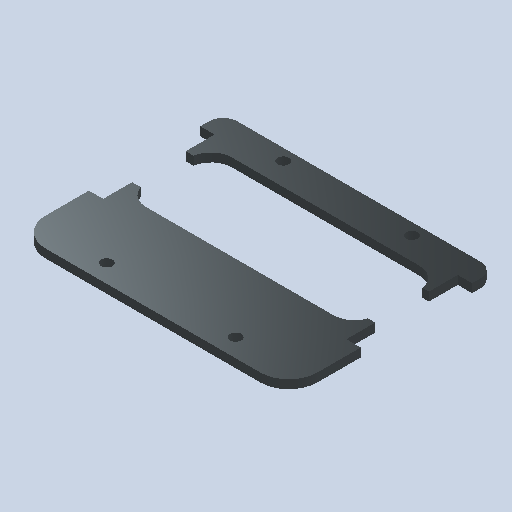
# Autodesk Inventor part: spacer
Saved by Autodesk Inventor 2022 (Build 260153000, 153)
## iProperties
Created: 2021-06-18
Part Number: spacer
Material: Iron, Gray
Document SubType Name: Modeling
Designer: benka
Density: 7.15 g/cm^3
Appearance: Iron Gray
Author: benka
Autodesk Inventor part; units mm, degrees
ref_plane "YZ Plane" through (0, 0, 0) normal (1, 0, 0) x (0, 1, 0)
ref_plane "XZ Plane" through (0, 0, 0) normal (0, 1, 0) x (-1, 0, 0)
ref_plane "XY Plane" through (0, 0, 0) normal (0, 0, 1) x (1, 0, 0)
sketch "Sketch1" plane through (0, 0, 0) normal (0, 1, 0) x (-1, 0, 0)
  arc A0 (-203.3189, -61.2561) -> (-210.2777, -66.3445) centre (-203.3189, -68.5586) ccw
  arc A1 (-130.8282, -66.3445) -> (-137.7869, -61.2561) centre (-137.7869, -68.5586) ccw
  arc A2 (-210.5383, -85.0627) -> (-203.3189, -91.2662) centre (-203.3189, -83.9637) ccw
  line L0 (-132.8206, -31.1315) -> (-207.8206, -31.1315)
  line L1 (-217.8206, -41.1315) -> (-217.8206, -56.2409)
  line L2 (-212.8206, -56.2409) -> (-217.8206, -56.2409) projected
  line L3 (-212.8206, -66.3445) -> (-212.8206, -56.2409) projected
  line L4 (-127.8206, -56.2409) -> (-127.8206, -66.3445) projected
  line L5 (-127.8206, -56.2409) -> (-122.8206, -56.2409) projected
  line L6 (-122.8206, -56.2409) -> (-122.8206, -41.1315)
  line L7 (-212.8206, -66.3445) -> (-210.2777, -66.3445)
  line L8 (-127.8206, -66.3445) -> (-130.8282, -66.3445)
  line L9 (-203.3189, -91.2662) -> (-137.7869, -91.2662)
  line L10 (-137.7869, -61.2561) -> (-203.3189, -61.2561) projected
  line L11 (-212.8208, -95.1662) -> (-212.8208, -85.0627) projected
  line L12 (-212.8208, -95.1662) -> (-217.8208, -95.1662) projected
  arc A3 (-217.8208, -98.1662) -> (-212.8208, -103.1662) centre (-212.8208, -98.1662) ccw projected
  arc A4 (-127.8208, -103.1662) -> (-122.8208, -98.1662) centre (-127.8208, -98.1662) ccw projected
  line L13 (-212.8208, -103.1662) -> (-127.8208, -103.1662)
  arc A5 (-137.7869, -91.2662) -> (-130.5676, -85.0627) centre (-137.7869, -83.9637) ccw
  line L14 (-217.8208, -98.1662) -> (-217.8208, -95.1662)
  line L15 (-212.8208, -85.0627) -> (-210.5383, -85.0627)
  line L16 (-127.8208, -95.1662) -> (-122.8208, -95.1662) projected
  line L17 (-127.8208, -85.0627) -> (-127.8208, -95.1662) projected
  line L18 (-127.8208, -85.0627) -> (-130.5676, -85.0627)
  line L19 (-122.8208, -98.1662) -> (-122.8208, -95.1662)
  circle A6 centre (-192.8208, -37.5164) radius 2 projected
  circle A7 centre (-147.8208, -37.5164) radius 2 projected
  circle A8 centre (-192.8208, -99.1662) radius 2 projected
  circle A9 centre (-147.8208, -99.1662) radius 2 projected
  arc A10 (-207.8206, -31.1315) -> (-217.8206, -41.1315) centre (-207.8206, -41.1315) ccw
  arc A11 (-122.8206, -41.1315) -> (-132.8206, -31.1315) centre (-132.8206, -41.1315) ccw
  point P0 (-122.8206, -31.1315)
  point P1 (-217.8206, -31.1315)
  point P2 (-189.2746, -36.1601)
  point P3 (-188.4494, -96.8743)
  dimension "d2" = 10
  constraints: 22 end point, 13 point on circle, 6 centre point, 5 point on line, 5 tangent, 2 horizontal, 2 perpendicular, 1 equal radius, 1 parallel, 2 other
  measures "d2" radius of A10
extrude "Extrusion1" add sketch "Sketch1" along normal blind 3
body "Solid1"
